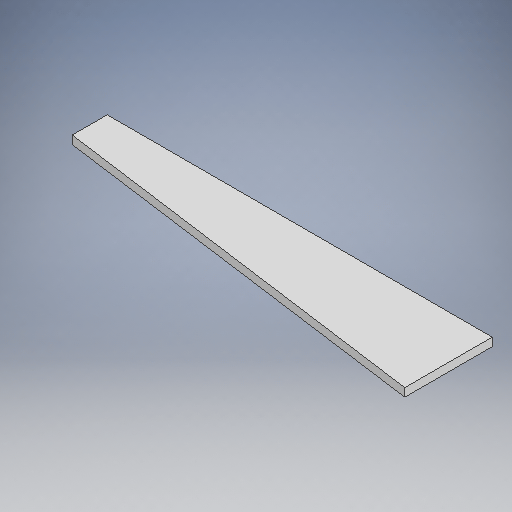
# Autodesk Inventor part: Mount_Support
Saved by Autodesk Inventor 2025.3 (Build 293356000, 356)
## iProperties
Created: 2025-12-10
Part Number: Mount_Support
Material: Generic
Document SubType Name: Modeling
Designer: sonata
Density: 1 g/cm^3
Appearance: Default
Author: sonata
Autodesk Inventor part; units mm, degrees
ref_plane "YZ Plane" through (0, 0, 0) normal (1, 0, 0) x (0, 1, 0)
ref_plane "XZ Plane" through (0, 0, 0) normal (0, 1, 0) x (-1, 0, 0)
ref_plane "XY Plane" through (0, 0, 0) normal (0, 0, 1) x (1, 0, 0)
sketch "Sketch1" plane through (0, 0, 0) normal (0, 1, 0) x (-1, 0, 0)
  line L0 (0, 0) -> (0, 25.4)
  line L1 (0, 0) -> (-279.4, 0)
  line L2 (-279.4, 0) -> (-279.4, 63.5)
  line L3 (0, 25.4) -> (-279.4, 63.5)
  dimension "d0" = 279.4
  dimension "d1" = 25.4
  dimension "d2" = 63.5
  constraints: 8 end point, 1 horizontal, 1 perpendicular, 1 vertical
  measures "d0" distance of L0.start L1.end
  measures "d1" distance of L0.start L0.end
  measures "d2" distance of L1.end L2.end
extrude "Extrusion1" add sketch "Sketch1" along normal blind 5.9995
sketch "Sketch2" plane through (279.4, 0, 0) normal (0, 0, -1) x (-1, 0, 0)
  line L0 (0, 0) -> (0, 5.9995) projected
  line L1 (279.4, 0) -> (279.4, 5.9995) projected
  line L2 (0, 0) -> (279.4, 0) projected
  point P0 (12.7, 2.9997)
  point P1 (76.2, 2.9997)
  point P2 (139.7, 2.9997)
  point P3 (203.2, 2.9997)
  point P4 (266.7, 2.9997)
  dimension "d5" = 12.7
  dimension "d6" = 12.7
  dimension "d7" = 2.9997
  dimension "d8" = 63.5
  dimension "d9" = 63.5
  dimension "d10" = 63.5
  dimension "d11" = 63.5
  constraints: 3 horizontal alignment
  measures "d5" distance from line of L0 point (12.7, 3)
  measures "d6" distance from line of L1 point (266.7, 3)
  measures "d7" distance from line of L2 point (266.7, 3)
  measures "d8" distance of point (76.2, 3) point (12.7, 3)
  measures "d9" distance of point (139.7, 3) point (76.2, 3)
  measures "d10" distance of point (203.2, 3) point (139.7, 3)
  measures "d11" distance of point (266.7, 3) point (203.2, 3)
hole "Hole1" at (266.7, 2.9997, 0) at (203.2, 2.9997, 0) at (139.7, 2.9997, 0) at (76.2, 2.9997, 0) at (12.7, 2.9997, 0) direction (0, 0, 1) diameter 2.6416 depth 19.05 thread size "6-32 UNC" class "2B" standard "ANSI Unified Screw Threads"
body "Solid1"
